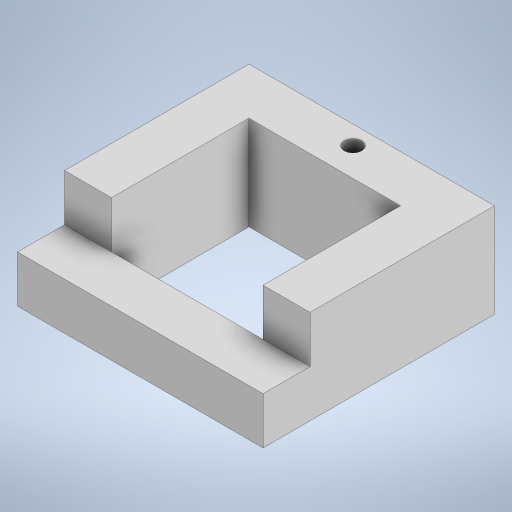
# Autodesk Inventor part: RJ45Adapter
Saved by Autodesk Inventor 2024 (Build 280153000, 153)
## iProperties
Created: 2025-09-21
Part Number: RJ45Adapter
Material: Generic
Document SubType Name: Modeling
Designer: Martin
Density: 1 g/cm^3
Appearance: Default
Author: Martin
Autodesk Inventor part; units mm, degrees
ref_plane "YZ Plane" through (0, 0, 0) normal (1, 0, 0) x (0, 1, 0)
ref_plane "XZ Plane" through (0, 0, 0) normal (0, 1, 0) x (-1, 0, 0)
ref_plane "XY Plane" through (0, 0, 0) normal (0, 0, 1) x (1, 0, 0)
sketch "Sketch1" plane through (0, 0, 0) normal (0, 1, 0) x (-1, 0, 0)
  line L0 (8.1915, 7.4295) -> (-8.1915, 7.4295)
  line L1 (-8.1915, 7.4295) -> (-8.1915, -7.4295)
  line L2 (-8.1915, -7.4295) -> (8.1915, -7.4295)
  line L3 (8.1915, -7.4295) -> (8.1915, 7.4295)
  line L4 (13.2715, -12.5095) -> (-13.2715, -12.5095)
  line L5 (-13.2715, -12.5095) -> (-13.2715, 12.5095)
  line L6 (-13.2715, 12.5095) -> (13.2715, 12.5095)
  line L7 (13.2715, 12.5095) -> (13.2715, -12.5095)
  point P0 (0, 0)
  point P1 (0, -7.4295)
  point P2 (8.1915, 0)
  dimension "d0" = 16.383
  dimension "d1" = 14.859
  dimension "d2" = 5.08
  constraints: 16 end point, 4 parallel, 2 midpoint, 2 perpendicular, 1 horizontal, 1 horizontal alignment, 1 vertical alignment, 3 other
  measures "d0" distance of L1.end L2.end
  measures "d1" distance of L0.end L1.end
  measures "d2" distance between parallel lines of L2 L4
extrude "Extrusion1" add sketch "Sketch1" along normal blind 5.08
sketch "Sketch2" plane through (0, 5.08, 0) normal (0, 1, 0) x (1, 0, 0)
  line L0 (-13.2715, -12.5095) -> (13.2715, -12.5095) projected
  line L1 (13.2715, -12.5095) -> (13.2715, 12.5095) projected
  line L2 (13.2715, 12.5095) -> (-13.2715, 12.5095) projected
  line L3 (-13.2715, 12.5095) -> (-13.2715, -12.5095) projected
  line L4 (-8.1915, -7.4295) -> (-8.1915, 7.4295) projected
  line L5 (-8.1915, 7.4295) -> (8.1915, 7.4295) projected
  line L6 (8.1915, 7.4295) -> (8.1915, -7.4295) projected
  line L7 (8.1915, -7.4295) -> (-8.1915, -7.4295) projected
  line L8 (-8.1915, -7.4295) -> (-13.2715, -7.4295)
  line L9 (8.1915, -7.4295) -> (-8.1915, -7.4295) projected
  line L10 (8.1915, -7.4295) -> (13.2715, -7.4295)
  point P0 (0, 0)
  constraints: 4 end point, 3 point on line, 1 horizontal
extrude "Extrusion2" add sketch "Sketch2" along normal blind 5.08 contours L3 L2 L1 L10 L6 L5 L4 L8
sketch "Sketch3" plane through (0, 10.16, 0) normal (0, 1, 0) x (1, 0, 0)
  line L0 (-8.1915, 7.4295) -> (8.1915, 7.4295) projected
  line L1 (-3.81, 7.4295) -> (3.81, 7.4295) construction
  line L2 (3.81, 7.4295) -> (3.81, 9.7155) construction
  line L3 (3.81, 9.7155) -> (-3.81, 9.7155) construction
  line L4 (-3.81, 9.7155) -> (-3.81, 7.4295) construction
  circle A0 centre (0, 10.4775) radius 1.143 construction
  circle A1 centre (0, 10.4775) radius 0.9525
  point P0 (0, 0)
  point P1 (0, 9.7155)
  point P2 (0, 7.4295)
  point P3 (0, 7.4295)
  dimension "d7" = 7.62
  dimension "d8" = 2.286
  dimension "d9" = 2.286
  dimension "d10" = 1.905
  dimension "d14" = 0.762
  constraints: 8 end point, 3 midpoint, 2 centre point, 2 parallel, 2 vertical alignment, 1 coincident, 1 horizontal, 1 perpendicular, 1 point on line
  measures "d7" distance of L3.end L2.end
  measures "d8" distance of L2.end L1.end
  measures "d9" diameter of A0
  measures "d10" diameter of A1
  measures "d14" distance of point (0, 9.716) A0.centre
extrude "Extrusion3" cut sketch "Sketch3" against normal blind 6.35
body "Solid1"
